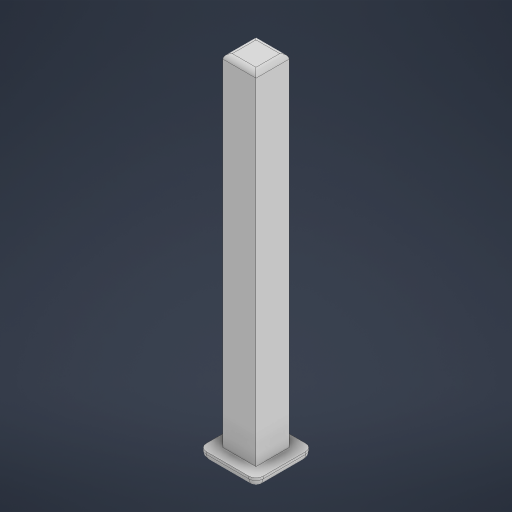
# Autodesk Inventor part: kołek
Saved by Autodesk Inventor 2024.4 (Build 284460000, 460)
## iProperties
Created: 2026-03-17
Part Number: kołek
Material: Ogólny
Document SubType Name: Modeling
Designer: User
Density: 1 g/cm^3
Appearance: Domyślna
Author: User
Autodesk Inventor part; units mm, degrees
ref_plane "YZ Plane" through (0, 0, 0) normal (1, 0, 0) x (0, 1, 0)
ref_plane "XZ Plane" through (0, 0, 0) normal (0, 1, 0) x (-1, 0, 0)
ref_plane "XY Plane" through (0, 0, 0) normal (0, 0, 1) x (1, 0, 0)
sketch "Szkic1" plane through (0, 0, 0) normal (0, 1, 0) x (-1, 0, 0)
  line L0 (-6, 6) -> (6, 6)
  line L1 (6, 6) -> (6, -6)
  line L2 (6, -6) -> (-6, -6)
  line L3 (-6, -6) -> (-6, 6)
  line L4 (-6, 6) -> (6, -6) construction
  line L5 (6, 6) -> (-6, -6) construction
  line L6 (-3.5, 3.5) -> (3.5, 3.5)
  line L7 (3.5, 3.5) -> (3.5, -3.5)
  line L8 (3.5, -3.5) -> (-3.5, -3.5)
  line L9 (-3.5, -3.5) -> (-3.5, 3.5)
  line L10 (-3.5, 3.5) -> (3.5, -3.5) construction
  line L11 (3.5, 3.5) -> (-3.5, -3.5) construction
  point P0 (0, 0)
  dimension "d0" = 12
  dimension "d1" = 12
  dimension "d2" = 7
  dimension "d3" = 7
  constraints: 24 end point, 4 midpoint, 4 parallel, 2 horizontal, 2 perpendicular
  measures "d0" distance of L1.end L2.end
  measures "d1" distance of L0.end L1.end
  measures "d2" distance of L7.end L8.end
  measures "d3" distance of L6.end L7.end
extrude "Wyciągnięcie proste1" add sketch "Szkic1" along normal blind 72 contours L6 L7 L8 L9
extrude "Wyciągnięcie proste2" add sketch "Szkic1" against normal blind 2 contours L0 L1 L2 L3 | L6 L7 L8 L9
fillet "Zaokrąglenie1" radius 1.5 8 edges at (6, -1, 6) (6, -1, -6) (-6, -1, 6) (-6, -1, -6) (0, -2, -6) (6, -2, 0) (0, -2, 6) (-6, -2, 0)
fillet "Zaokrąglenie2" radius 1 4 edges at (3.5, 72, 0) (0, 72, 3.5) (0, 72, -3.5) (-3.5, 72, 0)
